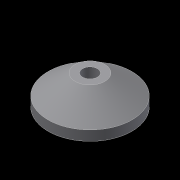
# Autodesk Inventor part: ForearmClampHead
Saved by Autodesk Inventor 2015 (Build 190159000, 159)
## iProperties
Created: 2014-10-19
Part Number: ForearmClampHead
Material: Generic
Document SubType Name: Modeling
Designer: Inventor
Mass: 0.858702 g
Surface Area: 6.50179 cm^2
Volume: 0.858702 cm^3
Density: 1 g/cm^3
Appearance: Default
Author: Inventor
Autodesk Inventor part; units mm, degrees
ref_plane "YZ Plane" through (0, 0, 0) normal (1, 0, 0) x (0, 1, 0)
ref_plane "XZ Plane" through (0, 0, 0) normal (0, 1, 0) x (-1, 0, 0)
sketch "Base" plane through (0, 0, 0) normal (0, 0, 1) x (1, 0, 0)
  circle A0 centre (0, 0) radius 8.5
  dimension "d0" = 17
  constraints: 1 centre point, 1 coincident
  measures "d0" diameter of A0
extrude "BaseFeature" add sketch "Base" along normal blind 2
sketch "LoftStart" plane through (0, 0, 2) normal (0, 0, 1) x (1, 0, 0)
  circle A0 centre (0, 0) radius 8.5 projected
ref_plane "LoftEndPlane" through (0, 0, 6) normal (0, 0, 1) x (1, 0, 0)
sketch "LoftEnd" plane through (0, 0, 6) normal (0, 0, 1) x (1, 0, 0)
  circle A0 centre (0, 0) radius 8.5 construction
  circle A1 centre (0, 0) radius 3
  dimension "d4" = 6
  constraints: 1 centre point, 1 coincident
  measures "d4" diameter of A1
loft "BellLoftFeature" add profiles "LoftStart", "LoftEnd"
sketch "TopHole" plane through (0, 0, 6) normal (0, 0, 1) x (1, 0, 0)
  circle A0 centre (0, 0) radius 3 projected
hole "TopHoleFeature" at (0, 0, 6) direction (0, 0, -1) diameter 3 end through all
body "Solid1"
